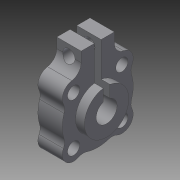
# Autodesk Inventor part: Clamping Hub
Saved by Autodesk Inventor 2014 SP1 (Build 180222100, 222)
## iProperties
Created: 2014-01-12
Part Number: Clamping Hub
Material: Generic
Document SubType Name: Modeling
Designer: tom
Density: 1 g/cm^3
Appearance: Default
Author: tom
Autodesk Inventor part; units mm, degrees
ref_plane "YZ Plane" through (0, 0, 0) normal (1, 0, 0) x (0, 1, 0)
ref_plane "XZ Plane" through (0, 0, 0) normal (0, 1, 0) x (-1, 0, 0)
ref_plane "XY Plane" through (0, 0, 0) normal (0, 0, 1) x (1, 0, 0)
sketch "Sketch1" plane through (0, 0, 0) normal (1, 0, 0) x (0, 1, 0)
  line L0 (-6.9148, -6.9148) -> (6.9148, 6.9148) construction
  circle A0 centre (0, 0) radius 9.779 construction
  line L1 (6.9148, -6.9148) -> (-7.1842, 7.1842) construction
  line L2 (0, 0) -> (9.779, 0) construction
  circle A1 centre (-6.9148, 6.9148) radius 1.7526
  circle A2 centre (6.9148, 6.9148) radius 1.7526
  circle A3 centre (-6.9148, -6.9148) radius 1.7526
  circle A4 centre (6.9148, -6.9148) radius 1.7526
  line L3 (-6.9148, -10.16) -> (-6.9148, 10.16) construction
  arc A5 (-5.4945, 9.8327) -> (-9.8327, 5.4945) centre (-6.9148, 6.9148) ccw
  arc A6 (-9.8327, -5.4945) -> (-5.4945, -9.8327) centre (-6.9148, -6.9148) ccw
  arc A7 (5.4945, -9.8327) -> (10.1186, -7.4317) centre (6.9148, -6.9148) ccw
  arc A8 (10.1186, 7.4317) -> (5.4945, 9.8327) centre (6.9148, 6.9148) ccw
  arc A9 (2.8448, 0.9525) -> (2.8405, -0.9652) centre (0, 0) ccw
  arc A10 (3.1276, 9.6666) -> (-3.1276, 9.6666) centre (0, 0) ccw
  line L4 (-10.16, 0) -> (16.129, 0) construction
  line L5 (16.129, 0.9525) -> (16.129, 4.7625) construction
  line L6 (16.129, -0.9652) -> (16.129, -4.7625) construction
  line L7 (16.129, 4.7625) -> (13.253, 4.7625)
  line L8 (16.129, -4.7625) -> (13.253, -4.7625)
  arc A11 (-9.6666, 3.1276) -> (-9.6666, -3.1276) centre (0, 0) ccw
  arc A12 (-3.1276, -9.6666) -> (3.1276, -9.6666) centre (0, 0) ccw
  line L9 (-10.16, -0.9652) -> (-10.114, -0.9652)
  line L10 (2.8405, -0.9652) -> (16.129, -0.9652)
  line L11 (-10.16, 0.9525) -> (-10.1153, 0.9525)
  line L12 (2.8448, 0.9525) -> (16.129, 0.9525)
  line L13 (16.129, 4.7625) -> (16.129, 0.9525)
  line L14 (16.129, -0.9652) -> (16.129, -4.7625)
  arc A13 (10.1186, 7.4317) -> (13.253, 4.7625) centre (13.253, 7.9375) ccw
  arc A14 (13.253, -4.7625) -> (10.1186, -7.4317) centre (13.253, -7.9375) ccw
  arc A15 (3.1276, 9.6666) -> (5.4945, 9.8327) centre (4.1049, 12.6875) ccw
  arc A16 (-5.4945, 9.8327) -> (-3.1276, 9.6666) centre (-4.1049, 12.6875) ccw
  arc A17 (-9.6666, 3.1276) -> (-9.8327, 5.4945) centre (-12.6875, 4.1049) ccw
  arc A18 (-9.8327, -5.4945) -> (-9.6666, -3.1276) centre (-12.6875, -4.1049) ccw
  arc A19 (-3.1276, -9.6666) -> (-5.4945, -9.8327) centre (-4.1049, -12.6875) ccw
  arc A20 (5.4945, -9.8327) -> (3.1276, -9.6666) centre (4.1049, -12.6875) ccw
  point P0 (9.3436, 4.7625)
  point P1 (9.3436, -4.7625)
  dimension "d4" = 19.558
  dimension "d6" = 3.5052
  dimension "d7" = 3.5052
  dimension "d8" = 3.5052
  dimension "d9" = 3.5052
  dimension "d11" = 6
  dimension "d12" = 26.289
  dimension "d18" = 3.175
  dimension "d19" = 3.175
  constraints: 42 point on circle, 30 end point, 21 centre point, 16 tangent, 6 coincident, 6 equal radius, 6 perpendicular, 5 parallel, 3 point on line, 1 collinear, 1 horizontal
  measures "d4" diameter of A0
  measures "d6" diameter of A1
  measures "d7" diameter of A2
  measures "d8" diameter of A3
  measures "d9" diameter of A4
  measures "d11" diameter of A9
  measures "d12" distance of L4.start L4.end
  measures "d18" radius of A13
  measures "d19" radius of A14
extrude "Extrusion1" add sketch "Sketch1" along normal blind 6.985
sketch "Sketch2" plane through (6.985, 0, 0) normal (1, 0, 0) x (0, 0, -1)
  line L0 (0.9652, 16.129) -> (0.9652, 2.8405) projected
  arc A0 (-0.9525, 2.8448) -> (0.9652, 2.8405) centre (0, 0) ccw projected
  line L1 (-0.9525, 2.8448) -> (-0.9525, 16.129) projected
  arc A1 (-0.9525, 6.2782) -> (0.9652, 6.2762) centre (0, 0) ccw
  arc A2 (-0.9525, 2.8448) -> (0.9652, 2.8405) centre (0, 0) ccw
  line L2 (-0.9525, 2.8448) -> (-0.9525, 6.2782)
  line L3 (0.9652, 2.8405) -> (0.9652, 6.2762)
  dimension "d22" = 12.7
  constraints: 4 end point, 4 point on circle, 2 centre point, 2 coincident, 2 point on line
  measures "d22" diameter of A1
extrude "Extrusion2" add sketch "Sketch2" along normal blind 2.54
sketch "Sketch3" plane through (0, 13.253, 4.7625) normal (0, 0, 1) x (1, 0, 0)
  line L0 (0, 0) -> (6.985, 0) projected
  circle A0 centre (3.4925, 0) radius 1.7526
  point P0 (0, -13.253)
  dimension "d25" = 3.5052
  constraints: 1 centre point, 1 midpoint
  measures "d25" diameter of A0
extrude "Extrusion3" cut sketch "Sketch3" along normal mid plane 29.5275
thread "Thread1" size "6-32 UNC" class "2B" standard "ANSI Unified Screw Threads" full length
thread "Thread2" size "6-32 UNC" class "2B" standard "ANSI Unified Screw Threads" full length
chamfer "Chamfer1" distance 0.254 angle 45 39 edges at (6.985, 11.1945, 5.5202) (6.985, 8.4102, 9.7949) (6.985, 4.3271, 9.5202) (6.985, 0, 10.16) (6.985, -4.3271, 9.5202) (6.985, -9.2095, 9.2095) (6.985, -9.5202, 4.3271) (6.985, -10.16, 0) (6.985, -9.5202, -4.3271) (6.985, -9.2095, -9.2095) (6.985, -4.3271, -9.5202) (6.985, 0, -10.16) (6.985, 4.3271, -9.5202) (6.985, 8.4102, -9.7949) (6.985, 11.1945, -5.5202) (6.985, 14.691, -4.7625) (6.985, 14.691, 4.7625) (0, 11.1945, 5.5202) (0, 8.4102, 9.7949) (0, 4.3271, 9.5202) (0, 0, 10.16) (0, -4.3271, 9.5202) (0, -9.2095, 9.2095) (0, -9.5202, 4.3271) (0, -10.16, 0) (0, -9.5202, -4.3271) (0, -9.2095, -9.2095) (0, -4.3271, -9.5202) (0, 0, -10.16) (0, 4.3271, -9.5202) (0, 8.4102, -9.7949) (0, 11.1945, -5.5202) (0, 14.691, -4.7625) (0, 14.691, 4.7625) (9.525, -6.35, 0.0064) (6.985, 16.129, -2.8638) (6.985, 16.129, 2.8575) (0, 16.129, -2.8638) (0, 16.129, 2.8575)
body "Solid1"
